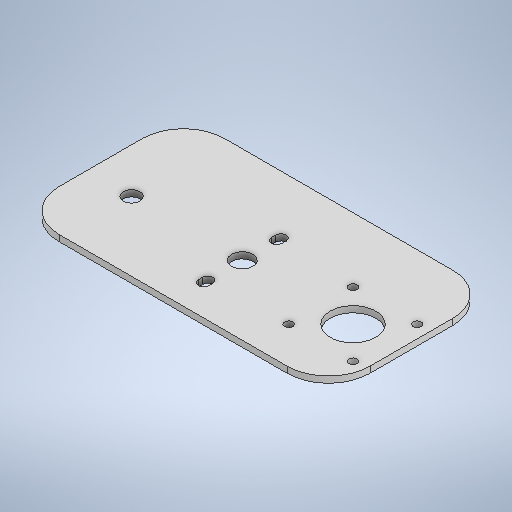
# Autodesk Inventor part: TopMount
Saved by Autodesk Inventor 2025.2 (Build 292293000, 293)
## iProperties
Created: 2025-07-18
Part Number: TopMount
Material: Generic
Document SubType Name: Modeling
Designer: Simon
Density: 1 g/cm^3
Appearance: Default
Author: Simon
Autodesk Inventor part; units mm, degrees
ref_plane "YZ Plane" through (0, 0, 0) normal (1, 0, 0) x (0, 1, 0)
ref_plane "XZ Plane" through (0, 0, 0) normal (0, 1, 0) x (-1, 0, 0)
ref_plane "XY Plane" through (0, 0, 0) normal (0, 0, 1) x (1, 0, 0)
sketch "Sketch1" plane through (0, 0, 0) normal (0, 1, 0) x (-1, 0, 0)
  line L0 (-75, 40) -> (75, 40)
  line L1 (75, 40) -> (75, -40)
  line L2 (75, -40) -> (-75, -40)
  line L3 (-75, -40) -> (-75, 40)
  line L4 (-75, 40) -> (75, -40) construction
  line L5 (75, 40) -> (-75, -40) construction
  point P0 (0, 0)
  dimension "d0" = 150
  dimension "d1" = 80
  constraints: 12 end point, 2 midpoint, 2 parallel, 1 horizontal, 1 perpendicular
  measures "d0" distance of L1.end L2.end
  measures "d1" distance of L0.end L1.end
extrude "Extrusion1" add sketch "Sketch1" along normal blind 3
sketch "Sketch5" plane through (0, 3, 0) normal (0, 1, 0) x (1, 0, 0)
  line L0 (-75, 40) -> (-75, -40) projected
  line L1 (75, 40) -> (-75, 40)
  line L2 (-75, 40) -> (-75, 15)
  line L3 (-75, 15) -> (75, 15)
  line L4 (75, 15) -> (75, 40)
  line L5 (21.6, 15) -> (-21.6, 15)
  line L6 (75, 15) -> (31.8, 15)
  line L7 (31.8, 15) -> (31.8, -28.2)
  line L8 (31.8, -28.2) -> (75, -28.2)
  line L9 (75, -28.2) -> (75, 15)
  line L10 (31.8, 15) -> (75, -28.2)
  line L11 (75, 15) -> (31.8, -28.2)
  circle A0 centre (53.4, -6.6) radius 11
  line L12 (37.9, -22.1) -> (68.9, -22.1)
  line L13 (68.9, -22.1) -> (68.9, 8.9)
  line L14 (68.9, 8.9) -> (37.9, 8.9)
  line L15 (37.9, 8.9) -> (37.9, -22.1)
  line L16 (37.9, -22.1) -> (68.9, 8.9) construction
  line L17 (68.9, -22.1) -> (37.9, 8.9) construction
  circle A1 centre (37.9, 8.9) radius 2
  circle A2 centre (68.9, 8.9) radius 2
  circle A3 centre (68.9, -22.1) radius 2
  circle A4 centre (37.9, -22.1) radius 2
  point P0 (309.988, -32.2194)
  dimension "d26" = 25
  dimension "d49" = 150
  dimension "d50" = 43.2
  dimension "d51" = 43.2
  dimension "d52" = 22
  dimension "d53" = 31
  dimension "d54" = 31
  dimension "d55" = 4
  dimension "d56" = 4
  dimension "d57" = 4
  dimension "d58" = 4
  constraints: 34 end point, 6 parallel, 5 centre point, 4 coincident, 3 horizontal, 3 midpoint, 3 perpendicular, 2 point on line
  measures "d26" distance of L2.end L1.end
  measures "d49" distance of L2.end L3.end
  measures "d50" distance of L8.end L7.end
  measures "d51" distance of L7.end L6.end
  measures "d52" diameter of A0
  measures "d53" distance of L14.end L13.end
  measures "d54" distance of L13.end L12.end
  measures "d55" diameter of A1
  measures "d56" diameter of A2
  measures "d57" diameter of A3
  measures "d58" diameter of A4
extrude "Extrusion4" cut sketch "Sketch5" against normal through all contours A2 L13 L11 | L11 L14 A2 | A1 L14 L10 | L10 L15 A1 | A3 L12 L10 | L10 L13 A3 | L13 A2 L11 | L11 A2 L14 | A4 L15 L11 | L11 L12 A4 | L14 A1 L10 | L10 A1 L15 | L12 A3 L10 | L10 A3 L13 | L15 A4 L11 | L11 A4 L12 | A0 L10 L11 | L11 L10 A0 | L10 L11 A0 | A0 L11 L10
sketch "Sketch6" plane through (0, 3, 0) normal (0, 1, 0) x (1, 0, 0)
  line L0 (75, 40) -> (-75, 40) projected
  line L1 (0, 40) -> (0, 15)
  line L2 (0, 15) -> (0, -28.2)
  line L3 (-21.6, 15) -> (21.6, 15)
  line L4 (21.6, 15) -> (21.6, -28.2)
  line L5 (21.6, -28.2) -> (-21.6, -28.2)
  line L6 (-21.6, -28.2) -> (-21.6, 15)
  line L7 (-21.6, 15) -> (21.6, -28.2) construction
  line L8 (21.6, 15) -> (-21.6, -28.2) construction
  circle A0 centre (0, -6.6) radius 5.1
  line L9 (0, 15) -> (75, 15)
  line L10 (75, 15) -> (31.8, 15)
  line L11 (31.8, 15) -> (31.8, -6.6)
  line L12 (31.8, -6.6) -> (53.4, -6.6)
  line L13 (53.4, -6.6) -> (0, -6.6)
  line L14 (0, -6.6) -> (-53.4, -6.6)
  circle A1 centre (-53.4, -6.6) radius 4
  line L15 (0, -25.25) -> (0, 12.05)
  circle A2 centre (0, 12.05) radius 2.5
  line L16 (0, 12.05) -> (0, 10.05)
  circle A3 centre (0, 10.05) radius 2.5
  circle A4 centre (0, -25.25) radius 2.5
  line L17 (0, -25.25) -> (0, -23.25)
  circle A5 centre (0, -23.25) radius 2.5
  line L18 (-2.5, -23.25) -> (-2.5, -25.25)
  line L19 (2.5, -23.25) -> (2.5, -25.25)
  line L20 (-2.5, 12.05) -> (-2.5, 10.05)
  line L21 (2.5, 12.05) -> (2.5, 10.05)
  point P0 (0, 0)
  dimension "d59" = 25
  dimension "d60" = 43.2
  dimension "d61" = 43.2
  dimension "d62" = 43.2
  dimension "d63" = 10.2
  dimension "d64" = 43.2
  dimension "d65" = 53.4
  dimension "d66" = 8
  dimension "d69" = 37.3
  dimension "d70" = 5
  dimension "d71" = 2
  dimension "d72" = 5
  dimension "d73" = 5
  dimension "d74" = 2
  dimension "d75" = 5
  constraints: 42 end point, 8 point on circle, 8 tangent, 7 point on line, 6 centre point, 6 coincident, 5 midpoint, 3 perpendicular, 2 parallel, 1 collinear, 1 horizontal, 1 vertical
  measures "d59" distance of L1.start L1.end
  measures "d60" distance of L1.end L2.end
  measures "d61" distance of L4.end L5.end
  measures "d62" distance of L3.end L4.end
  measures "d63" diameter of A0
  measures "d64" distance of L9.end L10.end
  measures "d65" distance of L13.end L14.end
  measures "d66" diameter of A1
  measures "d69" distance of L15.start L15.end
  measures "d70" diameter of A2
  measures "d71" distance of L16.start L16.end
  measures "d72" diameter of A3
  measures "d73" diameter of A4
  measures "d74" distance of L17.start L17.end
  measures "d75" diameter of A5
extrude "Extrusion6" cut sketch "Sketch6" against normal through all contours L2 A3 A2 | L2 A2 A3 | A3 A2 L2 | L2 A2 A3 | A2 A3 L2 | L2 A3 A2 | A2 L21 A3 | A3 L20 A2 | A1 | A0 L13 L2 | L2 L14 A0 | L13 A0 L2 | L2 A0 L14 | A5 A4 L2 | L2 A4 A5 | A4 A5 L2 | L2 A5 A4 | L19 A4 A5 | A5 A4 L18 | A4 A5 L2 | L2 A5 A4
fillet "Fillet1" radius 20 4 edges at (75, 1.5, 40) (75, 1.5, -40) (-75, 1.5, 40) (-75, 1.5, -40)
body "Solid1"
